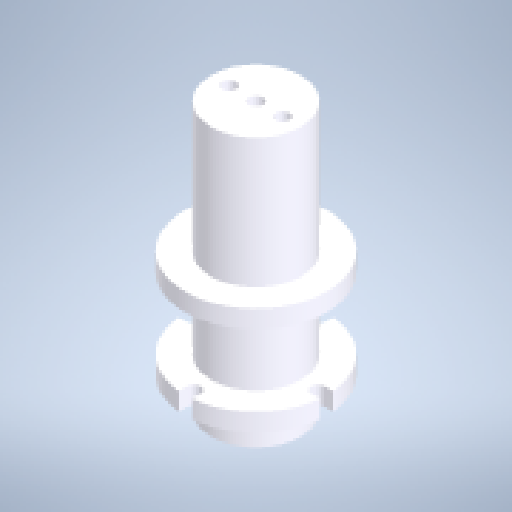
# Autodesk Inventor part: 033
Saved by Autodesk Inventor 2023 (Build 270158000, 158)
## iProperties
Created: 2022-04-13
Part Number: 033
Material: Glass
Document SubType Name: Modeling
Designer: Vinicius Miguel
Density: 2.18 g/cm^3
Appearance: Cool White
Author: Vinicius Miguel
Autodesk Inventor part; units mm, degrees
ref_plane "YZ Plane" through (0, 0, 0) normal (1, 0, 0) x (0, 1, 0)
ref_plane "XZ Plane" through (0, 0, 0) normal (0, 1, 0) x (-1, 0, 0)
ref_plane "XY Plane" through (0, 0, 0) normal (0, 0, 1) x (1, 0, 0)
sketch "Sketch5" plane through (0, 0, 0) normal (0, 0, 1) x (1, 0, 0)
  line L0 (0, 0) -> (0, 60)
  line L1 (0, 0) -> (10, 0)
  line L2 (10, 0) -> (10, 7)
  line L3 (10, 7) -> (15.85, 7)
  line L4 (15.85, 7) -> (15.85, 11)
  line L5 (15.85, 11) -> (10, 11)
  line L6 (10, 11) -> (10, 27)
  line L7 (10, 27) -> (15.85, 27)
  line L8 (15.85, 31) -> (10, 31)
  line L9 (10, 31) -> (10, 60)
  line L10 (10, 60) -> (0, 60)
  line L11 (15.85, 31) -> (15.85, 27)
  dimension "d17" = 31.7
  dimension "d18" = 7
  dimension "d19" = 4
  dimension "d23" = 20
  dimension "d26" = 60
  dimension "d27" = 20
  dimension "d48" = 31.7
  dimension "d49" = 16
  dimension "d50" = 4
  constraints: 24 end point, 8 perpendicular, 2 vertical, 2 vertical alignment, 1 horizontal
  measures "d17" diameter of L4 L0
  measures "d18" distance of L1.end L2.end
  measures "d19" distance of L3.end L4.end
  measures "d23" diameter of L6 L0
  measures "d26" distance of L0.start L0.end
  measures "d27" diameter of L2 L0
  measures "d48" diameter of L11 L0
  measures "d49" distance of L5.end L6.end
  measures "d50" distance of L8.start L7.end
revolve "Revolution1" add sketch "Sketch5" angle 360 about axis through (0, 0, 0) along (0, 1, 0)
sketch "Sketch6" plane through (0, 0, 0) normal (0, -1, 0) x (1, 0, 0)
  line L0 (-6, 0) -> (6, 0)
  point P0 (0, 0)
  point P1 (0, 0)
  point P2 (6, 0)
  point P3 (0, 0)
  point P4 (0, 0)
  dimension "d29" = 12
  constraints: 5 coincident, 2 end point, 1 horizontal, 1 midpoint
  measures "d29" distance of L0.start L0.end
hole "Hole2" at (0, 0, 0) at (6, 0, 0) at (-6, 0, 0) direction (0, 1, 0) diameter 3 end through all counterbore diameter 5 counterbore depth 10
sketch "Sketch7" plane through (0, 0, 0) normal (0, -1, 0) x (1, 0, 0)
  circle A0 centre (0, 0) radius 2.5 projected
  line L0 (-2.5, 0) -> (-2.5, -20)
  line L1 (-2.5, -20) -> (2.5, -20)
  line L2 (2.5, -20) -> (2.5, 0)
  point P0 (0, -20)
  dimension "d37" = 20
  constraints: 6 end point, 2 horizontal alignment, 2 point on circle, 1 midpoint, 1 perpendicular, 1 tangent, 1 vertical
  measures "d37" distance of point (0, -20) point (0, 0)
extrude "Extrusion4" cut sketch "Sketch7" against normal blind 8 contours L2 L1 L0 A0
sketch "Sketch8" plane through (0, 7, 0) normal (0, -1, 0) x (1, 0, 0)
  line L0 (-17.88, 0) -> (-13.88, 0) construction
  line L1 (-17.88, 1.5) -> (-13.88, 1.5)
  line L2 (-13.88, -1.5) -> (-17.88, -1.5)
  arc A0 (-17.88, 1.5) -> (-17.88, -1.5) centre (-17.88, 0) ccw
  arc A1 (-13.88, -1.5) -> (-13.88, 1.5) centre (-13.88, 0) ccw
  point P0 (0, 0)
  point P1 (-15.88, 0)
  dimension "d40" = 13.88
  dimension "d41" = 1.5
  dimension "d42" = 4
  constraints: 8 end point, 4 point on circle, 4 tangent, 2 centre point, 1 horizontal, 1 midpoint, 1 parallel
  measures "d40" distance of L0.end point (0, 0)
  measures "d41" radius of A0
  measures "d42" distance of L0.start L0.end
extrude "Extrusion5" cut sketch "Sketch8" against normal up to surface (4 mm away)
pattern_circular "Circular Pattern1" count 4 over 360 about axis through (0, 3.5, 0) along (0, 1, 0) of "Extrusion5"
body "Solid2"
